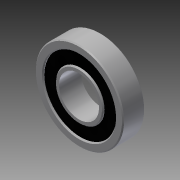
# Autodesk Inventor part: R10-2RS
Saved by Autodesk Inventor 2013 (Build 170138000, 138)
## iProperties
Created: 2013-06-05
Part Number: R10-2RS
Material: Generic
Document SubType Name: Modeling
Designer: mvarma
Density: 1 g/cm^3
Author: mvarma
Autodesk Inventor part; units mm, degrees
ref_plane "YZ Plane" through (0, 0, 0) normal (1, 0, 0) x (0, 1, 0)
ref_plane "XZ Plane" through (0, 0, 0) normal (0, 1, 0) x (-1, 0, 0)
ref_plane "XY Plane" through (0, 0, 0) normal (0, 0, 1) x (1, 0, 0)
sketch "Sketch1" plane through (0, 0, 0) normal (0, 0, 1) x (1, 0, 0)
  circle A0 centre (0, 0) radius 17.4625
  circle A1 centre (0, 0) radius 7.9375
  dimension "d0" = 34.925
  dimension "d2" = 15.875
  constraints: 2 centre point, 2 coincident
  measures "d0" diameter of A0
  measures "d2" diameter of A1
extrude "Extrusion1" add sketch "Sketch1" along normal blind 4.3656
sketch "Sketch2" plane through (0, 0, 4.3656) normal (0, 0, 1) x (1, 0, 0)
  circle A0 centre (0, 0) radius 17.4625 projected
  circle A1 centre (0, 0) radius 9.525
  circle A2 centre (0, 0) radius 14.2875
  dimension "d5" = 19.05
  dimension "d8" = 28.575
  constraints: 2 centre point, 2 coincident
  measures "d5" diameter of A1
  measures "d8" diameter of A2
extrude "Extrusion2" cut sketch "Sketch2" against normal blind 0.5953 contours A2
chamfer "Chamfer1" distance 0.3969 angle 45 3 edges at (-17.4625, 0, 4.3656) (-9.525, 0, 4.3656) (-14.2875, 0, 4.3656)
mirror "Mirror1" about plane through (0, 0, 0) normal (0, 0, -1)
body "Solid1"
